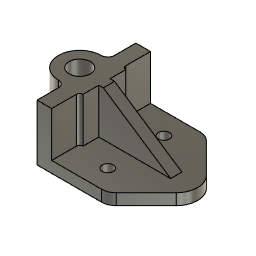
A3 (Autodesk Fusion 360 design; units mm, degrees)
Autodesk Fusion 360 part; units mm, degrees
sketch "Base" plane through (0, 0, 0) normal (0, 0, 1) x (1, 0, 0)
  line L0 (0, 0) -> (86, 0)
  line L1 (86, 0) -> (86, 88)
  line L2 (86, 88) -> (0, 88)
  line L3 (0, 88) -> (0, 0)
  line L4 (0, 0) -> (0, 88) construction
  line L5 (0, 44) -> (86, 44) construction
  circle A0 centre (67, 44) radius 19 construction
  line L6 (67, 44) -> (67, 25) construction
  line L7 (67, 44) -> (80.435, 30.565) construction
  line L8 (67, 44) -> (86, 44) construction
  line L9 (67, 44) -> (67, 63) construction
  line L10 (80.435, 30.565) -> (49.8701, 0)
  circle A1 centre (67, 44) radius 19
  line L11 (80.435, 57.435) -> (49.8701, 88)
  dimension "d1" = 86
  dimension "d2" = 88
  dimension "d3" = 38
  dimension "d4" = 45
  constraint horizontal L0
  constraint vertical L1
  constraint horizontal L2
  constraint vertical L3
  constraint coincident L0.start L3.end
  constraint midpoint L4 L5.start
  constraint midpoint L1 L5.end
  constraint coincident L5.end A0
  constraint coincident A0.centre L6.start
  constraint coincident A0 L6.end
  constraint perpendicular L5 L6
  constraint horizontal L8
  constraint coincident A0 L9.end
  constraint perpendicular L5 L9
  constraint coincident L0 L10.end
  constraint tangent A0 L10
  constraint coincident L5.end A1
  constraint tangent L1 A1
  constraint symmetric L5 L7.end L11.start
  constraint symmetric L5 L10.end L11.end
  measures "d1" distance of L0.start L0.end
  measures "d2" distance of L0.start L2.end
  measures "d3" diameter of A0
  measures "d4" angle of L7 L8
extrude "Extrude1" add sketch "Base" along normal blind 10 contours L0 L2 L3 L10 A1 L11 | A1
fillet "Fillet1" radius 13 2 edges at (49.8701, 0, 5) (49.8701, 88, 5)
sketch "First Body" plane through (0, 0, 10) normal (0, 0, 1) x (-1, 0, 0)
  arc A0 (-53.6777, -84.1924) -> (-44.4853, -88) centre (-44.4853, -75) ccw
  line L0 (-44.4853, -88) -> (0, -88)
  line L1 (0, -88) -> (0, 0)
  line L2 (0, 0) -> (-44.4853, 0)
  arc A1 (-44.4853, 0) -> (-53.6777, -3.8076) centre (-44.4853, -13) ccw
  line L3 (-53.6777, -3.8076) -> (-80.435, -30.565)
  arc A2 (-80.435, -30.565) -> (-80.435, -57.435) centre (-67, -44) ccw
  line L4 (-80.435, -57.435) -> (-53.6777, -84.1924)
  line L5 (0, 0) -> (13, 0)
  line L6 (13, 0) -> (13, -88)
  line L7 (13, -88) -> (0, -88)
  line L8 (0, -88) -> (0, 0)
  dimension "d10" = 13
  dimension "d11" = 88
  constraint horizontal L5
  constraint vertical L6
  constraint horizontal L7
  constraint vertical L8
  constraint coincident L1.end L2.start
  measures "d10" distance of L1.end L5.end
  measures "d11" distance of L1.end L0.end
extrude "Extrude2" add sketch "First Body" against normal blind 10 contours L1 L5 L6 L7 L8
sketch "First Body Extended" plane through (0, 0, 10) normal (0, 0, 1) x (-1, 0, 0)
  arc A0 (-53.6777, -84.1924) -> (-44.4853, -88) centre (-44.4853, -75) ccw
  line L0 (-44.4853, -88) -> (13, -88)
  line L1 (13, -88) -> (13, 0)
  line L2 (13, 0) -> (-44.4853, 0)
  arc A1 (-44.4853, 0) -> (-53.6777, -3.8076) centre (-44.4853, -13) ccw
  line L3 (-53.6777, -3.8076) -> (-80.435, -30.565)
  arc A2 (-80.435, -30.565) -> (-80.435, -57.435) centre (-67, -44) ccw
  line L4 (-80.435, -57.435) -> (-53.6777, -84.1924)
  line L5 (13, -88) -> (0, -88)
  line L6 (0, -88) -> (0, 0)
  line L7 (0, 0) -> (13, 0)
  line L8 (13, 0) -> (13, -88)
  line L9 (13, -88) -> (13, 0) construction
  line L10 (13, -44) -> (-85, -44) construction
  line L11 (13, -44) -> (13, -66)
  line L12 (13, -66) -> (-3, -66)
  line L13 (-3, -66) -> (-3, -44)
  line L14 (13, -44) -> (13, -22)
  line L15 (13, 0) -> (13, -88) construction
  line L16 (13, -22) -> (-3, -22)
  line L17 (-3, -22) -> (-3, -44)
  circle A3 centre (-3, -22) radius 3
  circle A4 centre (-3, -66) radius 3
  line L18 (-3, -44) -> (-3, -49)
  line L19 (-3, -49) -> (-7, -49)
  line L20 (-7, -49) -> (-7, -39)
  line L21 (-7, -39) -> (-3, -39)
  line L22 (-3, -39) -> (-3, -49)
  dimension "d14" = 13
  dimension "d15" = 88
  dimension "d18" = 22
  dimension "d19" = 16
  dimension "d20" = 22
  constraint horizontal L5
  constraint vertical L6
  constraint horizontal L7
  constraint vertical L8
  constraint coincident L0.end L1.start
  constraint midpoint L9 L10.start
  constraint perpendicular L9 L10
  constraint perpendicular L10 L11
  constraint perpendicular L6 L12
  constraint coincident L10 L13.end
  constraint perpendicular L10 L13
  constraint perpendicular L10 L14
  constraint symmetric L0.end L10 L1.end
  constraint symmetric L1.end L10 L0.end
  constraint symmetric L10 L11.end L14.end
  constraint symmetric L10 L12.end L16.end
  constraint symmetric L10 L13.end L17.end
  constraint coincident L16.end L17.start
  constraint tangent L6 A3
  constraint coincident L12.end L13.start
  constraint tangent L6 A4
  constraint coincident L13 L18.end
  constraint perpendicular L10 L18
  constraint perpendicular L13 L19
  constraint perpendicular L10 L20
  constraint coincident L17 L21.end
  constraint perpendicular L17 L21
  measures "d14" distance of L0.end L5.end
  measures "d15" distance of L0.end L1.end
  measures "d18" distance of L10.start L11.end
  measures "d19" distance of L11.end L12.end
  measures "d20" distance of L10.start L14.end
extrude "Extrude4" add sketch "First Body Extended" along normal blind 40 contours L0 L1 L5 L6 L8 L12 | L6 L13 L17 A3 A4 L18 L22 | L1 L6 L8 L11 L12 L14 L16 | L1 L2 L6 L7 L8 L16
extrude "Extrude5" add sketch "First Body Extended" along normal blind 40 contours L13 L17 L18 L19 L20 L21 L22
sketch "Triangle" plane through (0, 0, 0) normal (0, 1, 0) x (1, 0, 0)
  line L0 (86, -10, 0) -> (67, -10, 44) construction
  line L1 (67, -10, 44) -> (7, -50, 44)
  line L2 (7, -50, 44) -> (7, -10, 44)
  line L3 (67, -10, 44) -> (7, -10, 44)
extrude "Extrude6" add sketch "Triangle" along normal mid plane 10 contours L1 L2 L3 in plane through (0, 44, 0) normal (0, 1, 0)
sketch "Cirlces" plane through (0, 0, 10) normal (0, 0, 1) x (-1, 0, 0)
  line L0 (0, 0) -> (-30, 0) construction
  line L1 (0, 0) -> (-31, 0) construction
  line L2 (-31, 0) -> (-31, -19) construction
  circle A0 centre (-31, -19) radius 5 construction
  circle A1 centre (-31, -19) radius 5
  line L3 (13, -44) -> (-85, -44)
  circle A2 centre (-31, -69) radius 5
  dimension "d28" = 31
  dimension "d29" = 19
  constraint coincident L0.start L1.start
  constraint horizontal L0
  constraint parallel L0 L1
  constraint perpendicular L1 L2
  constraint coincident L2.end A0.centre
  constraint symmetric A1 L3 A2
  measures "d28" distance of L0.start L1.end
  measures "d29" distance of L1.end L2.end
extrude "Extrude7" cut sketch "Cirlces" against normal blind 37
sketch "Circles Back" plane through (0, 0, 50) normal (0, 0, 1) x (-1, 0, 0)
  line L0 (13, -88) -> (13, 0)
  line L1 (13, 0) -> (0, 0)
  line L2 (0, 0) -> (0, -22)
  arc A0 (-3, -25) -> (0, -22) centre (-3, -22) ccw
  line L3 (-3, -25) -> (-3, -39)
  line L4 (-3, -39) -> (-7, -39)
  line L5 (-7, -39) -> (-7, -49)
  line L6 (-7, -49) -> (-3, -49)
  line L7 (-3, -49) -> (-3, -63)
  arc A1 (0, -66) -> (-3, -63) centre (-3, -66) ccw
  line L8 (0, -66) -> (0, -88)
  line L9 (0, -88) -> (13, -88)
  line L10 (13, -44) -> (13, -63)
  line L11 (13, -44) -> (13, -25)
  line L12 (13, -25) -> (25, -25)
  line L13 (25, -25) -> (25, -13)
  line L14 (25, -13) -> (13, -13)
  line L15 (13, -13) -> (13, -25)
  circle A2 centre (19, -19) radius 6
  line L16 (13, -44) -> (-26, -44) construction
  circle A3 centre (19, -69) radius 6
  line L17 (13, -63) -> (25, -63)
  line L18 (25, -63) -> (25, -75)
  line L19 (25, -75) -> (13, -75)
  circle A4 centre (19, -44) radius 19 construction
  circle A5 centre (19, -44) radius 19
  circle A6 centre (19, -44) radius 9.5
  dimension "d49" = 19
  dimension "d50" = 19
  dimension "d51" = 12
  dimension "d52" = 12
  dimension "d53" = 19
  constraint midpoint L0 L10.start
  constraint parallel L0 L10
  constraint parallel L0 L11
  constraint horizontal L12
  constraint vertical L13
  constraint horizontal L14
  constraint vertical L15
  constraint tangent L15 A2
  constraint perpendicular L10 L16
  constraint symmetric L11.end L16 L10.end
  constraint symmetric L12.end L16 L17.end
  constraint symmetric L13.end L16 L18.end
  constraint symmetric L14.end L16 L19.end
  constraint symmetric A2 L16 A3
  constraint tangent A2 A4
  constraint tangent A2 A5
  constraint concentric A5 A6
  measures "d49" distance of L10.start L10.end
  measures "d50" distance of L10.start L11.end
  measures "d51" distance of L11.end L12.end
  measures "d52" distance of L11.end L14.end
  measures "d53" diameter of A6
extrude "Extrude13" cut sketch "Circles Back" against normal blind 78 contours L0 L10 L11 A6 picked at (10.7012, -43.5335)
extrude "Extrude12" add sketch "Circles Back" against normal blind 50 contours L0 A3 L17 | L0 L10 L17 A5 | L0 L10 L11 A5 A6 | L0 L10 L11 A5 A6 | L0 L11 L12 A5 | L0 L12 L15 A2
sketch "Back Circle" plane through (0, 0, 50) normal (0, 0, 1) x (-1, 0, 0)
  line L0 (13, -88) -> (13, 0)
  line L1 (13, 0) -> (0, 0)
  line L2 (0, 0) -> (0, -22)
  arc A0 (-3, -25) -> (0, -22) centre (-3, -22) ccw
  line L3 (-3, -25) -> (-3, -39)
  line L4 (-3, -39) -> (-7, -39)
  line L5 (-7, -39) -> (-7, -49)
  line L6 (-7, -49) -> (-3, -49)
  line L7 (-3, -49) -> (-3, -63)
  arc A1 (0, -66) -> (-3, -63) centre (-3, -66) ccw
  line L8 (0, -66) -> (0, -88)
  line L9 (0, -88) -> (13, -88)
  line L10 (-3, -63) -> (35, -63)
  line L11 (35, -63) -> (35, -25)
  line L12 (35, -25) -> (-3, -25)
  line L13 (-3, -25) -> (-3, -63)
  circle A2 centre (16, -44) radius 19
  circle A3 centre (16, -44) radius 9.5
  line L14 (13, -25) -> (25, -25)
  line L15 (13, -13) -> (13, -25)
  line L16 (13, -44) -> (-85, -44)
  line L17 (13, -75) -> (13, -63)
  line L18 (13, -63) -> (25, -63)
  line L19 (13, -25) -> (19, -25)
  line L20 (19, -25) -> (19, -19)
  line L21 (19, -19) -> (13, -19)
  line L22 (13, -19) -> (13, -25)
  line L23 (13, -63) -> (19, -63)
  line L24 (19, -63) -> (19, -69)
  line L25 (19, -69) -> (13, -69)
  line L26 (13, -69) -> (13, -63)
  dimension "d32" = 38
  dimension "d33" = 38
  dimension "d34" = 19
  dimension "d35" = 12
  dimension "d36" = 12
  dimension "d43" = 6
  dimension "d44" = 6
  dimension "d45" = 6
  dimension "d46" = 6
  constraint horizontal L10
  constraint vertical L11
  constraint horizontal L12
  constraint vertical L13
  constraint coincident L7.end A1.end
  constraint tangent L13 A2
  constraint concentric A2 A3
  constraint horizontal L14
  constraint vertical L15
  constraint coincident L12 L14.start
  constraint coincident L0 L14.start
  constraint symmetric L14.start L16 L17.end
  constraint symmetric L14.end L16 L18.end
  constraint symmetric L15.start L16 L17.start
  constraint horizontal L19
  constraint vertical L20
  constraint horizontal L21
  constraint vertical L22
  constraint horizontal L23
  constraint vertical L24
  constraint horizontal L25
  constraint vertical L26
  measures "d32" distance of L7.end L10.end
  measures "d33" distance of L7.end A0.start
  measures "d34" diameter of A3
  measures "d35" distance of L14.start L14.end
  measures "d36" distance of L14.start L15.start
  measures "d43" distance of L14.start L21.end
  measures "d44" distance of L14.start L19.end
  measures "d45" distance of L17.end L23.end
  measures "d46" distance of L17.end L25.end
extrude "Extrude11" [suppressed]
extrude "Extrude10" [suppressed]
extrude "Extrude9" [suppressed]
extrude "Extrude8" [suppressed]
extrude "Extrude3" [suppressed]
equation "d3 = ( 19 * 2 ) * 1 mm"
equation "d18 = ( ( 38 + 6 ) / 2 ) * 1 mm"
equation "d19 = 13 mm + 3 mm"
equation "d29 = ( 38 / 2 ) * 1 mm"
equation "d49 = ( 38 / 2 ) * 1 mm"
named bodies: "Object"
